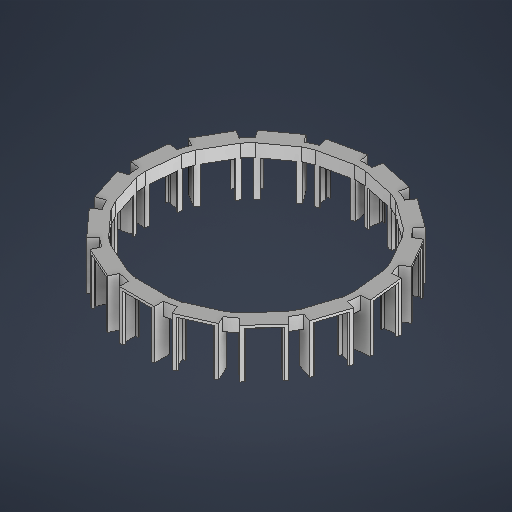
# Autodesk Inventor part: Sphere_V2
Saved by Autodesk Inventor 2025.1 (Build 291241020, 241B)
## iProperties
Created: 2024-09-22
Part Number: Sphere_V2
Material: Generic
Document SubType Name: Modeling
Designer: Sora
Density: 1 g/cm^3
Appearance: Default
Author: Sora
Autodesk Inventor part; units mm, degrees
ref_plane "YZ Plane" through (0, 0, 0) normal (1, 0, 0) x (0, 1, 0)
ref_plane "XZ Plane" through (0, 0, 0) normal (0, 1, 0) x (-1, 0, 0)
ref_plane "XY Plane" through (0, 0, 0) normal (0, 0, 1) x (1, 0, 0)
sketch "Sketch1" plane through (0, 0, 0) normal (0, 1, 0) x (-1, 0, 0)
  circle A0 centre (0, 0) radius 81
  circle A1 centre (0, 0) radius 86
  dimension "d0" = 162
  dimension "d1" = 5
  constraints: 2 centre point, 1 coincident
  measures "d0" diameter of A0
  measures "d1" radial gap between concentric circles of A0 A1
extrude "Extrusion1" add sketch "Sketch1" along normal blind 10
sketch "Sketch3" plane through (0, 10, 0) normal (0, 1, 0) x (1, 0, 0)
  circle A0 centre (0, 0) radius 86 projected
  line L0 (-13.5, -80) -> (13.5, -80)
  line L1 (13.5, -80) -> (13.5, -92)
  line L2 (13.5, -92) -> (-13.5, -92)
  line L3 (-13.5, -92) -> (-13.5, -80)
  line L4 (-13.5, -80) -> (13.5, -92) construction
  line L5 (13.5, -80) -> (-13.5, -92) construction
  line L6 (0, 0) -> (0, -86)
  point P0 (13.5, -84.9338)
  point P1 (-13.5, -84.9338)
  dimension "d4" = 27
  dimension "d5" = 12
  constraints: 14 end point, 2 midpoint, 2 parallel, 1 horizontal, 1 perpendicular, 1 vertical, 2 other
  measures "d4" distance of L1.end L2.end
  measures "d5" distance of L0.end L1.end
extrude "Extrusion2" add sketch "Sketch3" against normal blind 38 contours L3 L0 L6 A0 | A0 L1 L2 L3 | A0 L6 L0 L1
sketch "Sketch4" plane through (0, -28, 0) normal (0, -1, 0) x (1, 0, 0)
  line L0 (13.5, 80) -> (13.5, 92) projected
  line L1 (13.5, 92) -> (-13.5, 92) projected
  line L2 (-13.5, 92) -> (-13.5, 80) projected
  line L3 (-13.5, 80) -> (13.5, 80) projected
  line L4 (0, 80) -> (0, 92) construction
  line L5 (-12.5, 89.1) -> (12.5, 89.1)
  line L6 (12.5, 89.1) -> (12.5, 91)
  line L7 (12.5, 91) -> (-12.5, 91)
  line L8 (-12.5, 91) -> (-12.5, 89.1)
  line L9 (-12.5, 89.1) -> (12.5, 91) construction
  line L10 (12.5, 89.1) -> (-12.5, 91) construction
  line L11 (-12, 81) -> (12, 81)
  line L12 (12, 81) -> (12, 89.1)
  line L13 (12, 89.1) -> (-12, 89.1)
  line L14 (-12, 89.1) -> (-12, 81)
  line L15 (-12, 81) -> (12, 89.1) construction
  line L16 (12, 81) -> (-12, 89.1) construction
  line L17 (-10, 91) -> (10, 91)
  line L18 (10, 91) -> (10, 92)
  line L19 (10, 92) -> (-10, 92)
  line L20 (-10, 92) -> (-10, 91)
  line L21 (-10, 91) -> (10, 92) construction
  line L22 (10, 91) -> (-10, 92) construction
  line L23 (-10, 81) -> (10, 81)
  line L24 (10, 81) -> (10, 80)
  line L25 (10, 80) -> (-10, 80)
  line L26 (-10, 80) -> (-10, 81)
  line L27 (-10, 81) -> (10, 80) construction
  line L28 (10, 81) -> (-10, 80) construction
  point P0 (0, 0)
  point P1 (0, 90.05)
  point P2 (0, 85.05)
  point P3 (0, 91.5)
  point P4 (0, 80.5)
  dimension "d8" = 25
  dimension "d9" = 1.9
  dimension "d10" = 1
  dimension "d11" = 24
  dimension "d12" = 1
  dimension "d13" = 20
  dimension "d22" = 20
  constraints: 50 end point, 10 midpoint, 8 parallel, 6 point on line, 4 horizontal, 4 perpendicular, 3 collinear
  measures "d8" distance of L7.end L6.end
  measures "d9" distance of L6.end L5.end
  measures "d10" distance between parallel lines of L1 L7
  measures "d11" distance of L13.end L12.end
  measures "d12" distance between parallel lines of L3 L11
  measures "d13" distance of L17.start L17.end
  measures "d22" distance of L23.start L23.end
extrude "Extrusion3" cut sketch "Sketch4" against normal blind 36 contours L18 L7 L20 L1 | L11 L14 L5 L12 | L7 L6 L5 L8
extrude "Extrusion4" cut sketch "Sketch4" against normal blind 28 contours L3 L26 L11 L24
chamfer "Chamfer1" distance 1 angle 45 2 edges at (10, -10, 92) (-10, -10, 92)
pattern_circular "Circular Pattern1" count 15 over 360 about axis through (0, -10, 0) along (0, 1, 0) of "Extrusion2", "Extrusion3", "Chamfer1", "Extrusion4"
equation "\"d22\" = d13"
body "Solid1"
